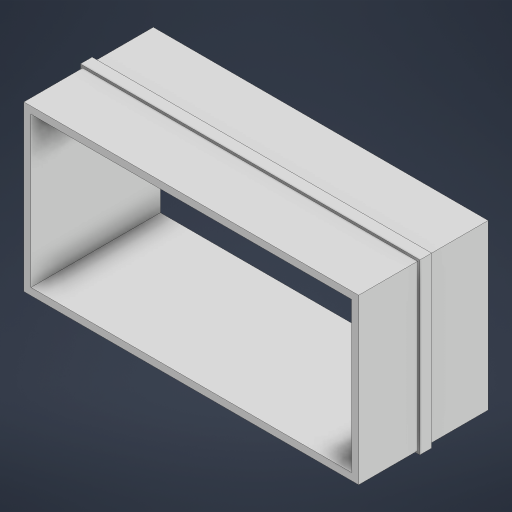
# Autodesk Inventor part: Connector
Saved by Autodesk Inventor 2024.2 (Build 282272000, 272)
## iProperties
Created: 2024-06-02
Part Number: Connector
Material: Generic
Document SubType Name: Modeling
Designer: simon
Density: 1 g/cm^3
Appearance: Default
Author: simon
Autodesk Inventor part; units mm, degrees
ref_plane "YZ Plane" through (0, 0, 0) normal (1, 0, 0) x (0, 1, 0)
ref_plane "XZ Plane" through (0, 0, 0) normal (0, 1, 0) x (-1, 0, 0)
ref_plane "XY Plane" through (0, 0, 0) normal (0, 0, 1) x (1, 0, 0)
sketch "Sketch1" plane through (0, 0, 0) normal (0, 0, 1) x (1, 0, 0)
  line L0 (0, 0) -> (56.9, 0)
  line L1 (56.9, 0) -> (56.9, 27.9)
  line L2 (56.9, 27.9) -> (0, 27.9)
  line L3 (0, 27.9) -> (0, 0)
  line L4 (1.2, 26.7) -> (55.7, 26.7)
  line L5 (55.7, 26.7) -> (55.7, 1.2)
  line L6 (55.7, 1.2) -> (1.2, 1.2)
  line L7 (1.2, 1.2) -> (1.2, 26.7)
  dimension "d0" = 56.9
  dimension "d1" = 27.9
  dimension "d2" = 1.2
  dimension "d3" = 1.2
  dimension "d4" = 1.2
  dimension "d5" = 1.2
  constraints: 16 end point, 4 parallel, 2 horizontal, 2 perpendicular
  measures "d0" distance of L2.end L1.end
  measures "d1" distance of L1.end L0.end
  measures "d2" distance between parallel lines of L2 L4
  measures "d3" distance between parallel lines of L3 L7
  measures "d4" distance between parallel lines of L0 L6
  measures "d5" distance between parallel lines of L1 L5
extrude "Extrusion1" add sketch "Sketch1" along normal blind 10
sketch "Sketch3" plane through (0, 0, 10) normal (0, 0, 1) x (1, 0, 0)
  line L0 (1.2, 26.7) -> (55.7, 26.7) projected
  line L1 (55.7, 26.7) -> (55.7, 1.2) projected
  line L2 (1.2, 26.7) -> (55.7, 26.7)
  line L3 (55.7, 26.7) -> (55.7, 1.2)
  line L4 (55.7, 1.2) -> (1.2, 1.2)
  line L5 (1.2, 1.2) -> (1.2, 26.7)
  line L6 (-0.4, 28.3) -> (57.3, 28.3)
  line L7 (57.3, 28.3) -> (57.3, -0.4)
  line L8 (57.3, -0.4) -> (-0.4, -0.4)
  line L9 (-0.4, -0.4) -> (-0.4, 28.3)
  point P0 (0, 0)
  dimension "d8" = 1.6
  dimension "d9" = 1.6
  dimension "d10" = 1.6
  dimension "d11" = 1.6
  constraints: 16 end point, 4 parallel, 2 horizontal, 2 perpendicular
  measures "d8" distance between parallel lines of L9 L5
  measures "d9" distance between parallel lines of L6 L0
  measures "d10" distance between parallel lines of L4 L8
  measures "d11" distance between parallel lines of L7 L1
extrude "Extrusion2" add sketch "Sketch3" along normal blind 2
sketch "Sketch4" plane through (0, 0, 12) normal (0, 0, 1) x (1, 0, 0)
  line L0 (1.2, 26.7) -> (55.7, 26.7) projected
  line L1 (55.7, 26.7) -> (55.7, 1.2) projected
  line L2 (1.2, 26.7) -> (55.7, 26.7)
  line L3 (55.7, 26.7) -> (55.7, 1.2)
  line L4 (55.7, 1.2) -> (1.2, 1.2)
  line L5 (1.2, 1.2) -> (1.2, 26.7)
  line L6 (56.9, 27.9) -> (0, 27.9) projected
  line L7 (56.9, 0) -> (56.9, 27.9) projected
  line L8 (0, 27.9) -> (56.9, 27.9)
  line L9 (56.9, 27.9) -> (56.9, 0)
  line L10 (56.9, 0) -> (0, 0)
  line L11 (0, 0) -> (0, 27.9)
  constraints: 16 end point, 4 parallel, 2 horizontal, 2 perpendicular
extrude "Extrusion3" add sketch "Sketch4" along normal blind 10
body "Solid1"
